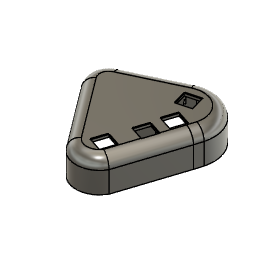
keyboard enclosure v1 (Autodesk Fusion 360 design; units mm, degrees)
Autodesk Fusion 360 part; units mm, degrees
note: some values were not read from the file. Set by a fixed rule: which face or edge a step refers to.
sketch "Sketch1" plane through (0, 0, 0) normal (0, 1, 0) x (1, 0, 0)
  line L0 (37.3318, 32.24) -> (56.8536, -27.823)
  line L1 (15.147, -72.2088) -> (-33.9094, -49.1235)
  line L2 (-42, -21) -> (0, 35)
  arc A0 (37.3318, 32.24) -> (0, 35) centre (17.782, 21.6635) ccw
  line L3 (-38.7396, -23.3195) -> (3.2, 32.6)
  arc A1 (33.646, 30.6398) -> (3.2, 32.6) centre (17.782, 21.6635) ccw
  line L4 (33.646, 30.6398) -> (53.0495, -29.0594)
  line L5 (18.0933, -69.1745) -> (-33.135, -45.0672)
  arc A2 (-38.7396, -23.3195) -> (-33.135, -45.0672) centre (-27.2324, -31.95) ccw
  arc A3 (-42, -21) -> (-33.9094, -49.1235) centre (-27.3274, -32.0045) ccw
  arc A4 (18.0933, -69.1745) -> (55.1557, -35.5397) centre (29.6328, -44.6529) ccw
  arc A5 (15.147, -72.2088) -> (59.1557, -35.5327) centre (28.6034, -43.6139) ccw
  line L6 (56.8536, -27.823) -> (59.1557, -35.5327)
  line L7 (53.0495, -29.0594) -> (55.1557, -35.5397)
  line L8 (52.453, -53.0201) -> (43.8544, -53.0201) construction
  line L9 (43.8544, -53.0201) -> (43.8544, -43.0201) construction
  line L10 (43.8544, -43.0201) -> (52.453, -43.0201) construction
  line L11 (52.453, -43.0201) -> (52.453, -53.0201) construction
  line L12 (17.453, -53.0201) -> (26.0516, -53.0201) construction
  line L13 (26.0516, -53.0201) -> (26.0516, -43.0201) construction
  line L14 (26.0516, -43.0201) -> (17.453, -43.0201) construction
  line L15 (17.453, -43.0201) -> (17.453, -53.0201) construction
  line L16 (19.8928, 4.2595) -> (7.5092, -13.426) construction
  line L17 (7.5092, -13.426) -> (-13.2972, 1.1429) construction
  line L18 (-13.2972, 1.1429) -> (-0.9137, 18.8283) construction
  line L19 (-0.9137, 18.8283) -> (19.8928, 4.2595) construction
  circle A6 centre (-0.9137, 18.8283) radius 1.25
  circle A7 centre (19.8928, 4.2595) radius 1.25
  circle A8 centre (-13.2972, 1.1429) radius 1.25
  circle A9 centre (7.5092, -13.426) radius 1.25
  point P0 (20.4966, 21.6635)
  point P1 (31.9109, -7.9188)
  point P2 (37.3318, -27.3652)
  point P3 (27.6914, -52.5189)
  point P4 (17.5, 42)
  point P5 (47.0927, -4.6835)
  point P6 (33.5812, -73.0892)
  point P7 (-42.8158, -37.0751)
  dimension "d55" = 4
  dimension "d56" = 4
  dimension "d70" = 21.59
  dimension "d71" = 25.4
  dimension "d72" = 2.5
  dimension "d73" = 2.5
  dimension "d74" = 2.5
  dimension "d75" = 2.5
  text T0 "v1" font "Arial" height 10 align ink ink in box 0 x 0 at (52.453, -53.0201) x (-1, 0) y (0, 1) spacing 1 kerned height is em
  text T1 "v1" font "Arial" height 10 align ink ink in box 0 x 0 at (17.453, -53.0201) x (1, 0) y (0, 1) spacing 1 height is em
  constraint tangent L2 A0
  constraint parallel L2 L3
  constraint concentric A0 A1
  constraint parallel L0 L4
  constraint tangent L3 A1
  constraint tangent L3 A2
  constraint tangent L2 A3
  constraint tangent L5 A4
  constraint tangent L1 A5
  constraint parallel L4 L7
  constraint perpendicular L8 L9
  constraint parallel L8 L10
  constraint parallel L9 L11
  constraint perpendicular L12 L13
  constraint parallel L12 L14
  constraint parallel L13 L15
  constraint coincident L18.end L19.start
  constraint coincident L16.start L19.end
  constraint coincident L17.end L18.start
  constraint coincident L16.end L17.start
  measures "d55" distance of L1 L5
  measures "d56" distance of A4.end A5.end
  measures "d70" distance of L16.start L16.end
  measures "d71" distance of L16.start L18.end
  measures "d72" diameter of A6
  measures "d73" diameter of A7
  measures "d74" diameter of A8
  measures "d75" diameter of A9
extrude "Extrude1" add sketch "Sketch1" along normal blind 30 contours L0 L1 L2 A0 A3 A5 L6 | L3 A1 L4 L5 A2 A4 L7 | A6 | A7 | A8 | A9 makes body 1
sketch "Sketch2" plane through (-25.0736, 0, 53.2816) normal (-0.425796, 0, 0.904819) x (0.904819, 0, 0.425796)
  line L0 (-9.7653, 0) -> (44.4515, 0)
  line L1 (44.4515, 30) -> (-9.7653, 30)
  line L2 (-7.9037, 17.6353) -> (-7.0737, 17.6353) construction
  line L3 (2.6065, 7.5699) -> (2.6065, 6.7399) construction
  line L4 (6.9063, 17.6353) -> (7.7363, 17.6353) construction
  line L5 (-7.0737, 7.5699) -> (-7.0737, 21.5499)
  line L6 (7.7363, 6.7399) -> (-7.9037, 6.7399)
  line L7 (-7.9037, 22.3799) -> (7.7363, 22.3799)
  line L8 (6.9063, 7.5699) -> (-7.0737, 7.5699)
  line L9 (6.9063, 21.5499) -> (6.9063, 7.5699)
  line L10 (7.7363, 22.3799) -> (7.7363, 6.7399)
  line L11 (-7.0737, 21.5499) -> (6.9063, 21.5499)
  line L12 (1.5152, 22.3799) -> (1.5152, 21.5499) construction
  line L13 (-7.9037, 6.7399) -> (-7.9037, 22.3799)
  line L14 (44.4515, 0) -> (44.4515, 30)
  line L15 (-9.7653, 30) -> (-9.7653, 0)
  point P0 (0, 15)
  dimension "d46" = 13.98
  dimension "d47" = 13.98
  dimension "d48" = 15.64
  dimension "d49" = 15.64
  constraint horizontal L11
  constraint vertical L9
  constraint horizontal L8
  constraint vertical L5
  constraint horizontal L7
  constraint vertical L10
  constraint horizontal L6
  constraint vertical L13
  constraint coincident L12.start L7
  constraint coincident L12.end L11
  constraint perpendicular L11 L12
  constraint coincident L3.start L8
  constraint coincident L3.end L6
  constraint perpendicular L3 L6
  constraint equal L3 L12
  constraint coincident L2.start L13
  constraint coincident L2.end L5
  constraint perpendicular L2 L5
  constraint coincident L4.start L9
  constraint coincident L4.end L10
  constraint perpendicular L4 L10
  constraint equal L2 L4
  measures "d46" distance of L5.end L9.start
  measures "d47" distance of L5.end L5.start
  measures "d48" distance of L6.end L7.start
  measures "d49" distance of L7.start L7.end
sketch "Sketch3" plane through (0, 0, 0) normal (0, 1, 0) x (1, 0, 0)
  line L0 (196.83, 143.17) -> (210.81, 143.17)
  line L1 (210.81, 143.17) -> (210.81, 129.19)
  line L2 (210.81, 129.19) -> (196.83, 129.19)
  line L3 (196.83, 129.19) -> (196.83, 143.17)
  line L4 (196, 144) -> (211.64, 144)
  line L5 (211.64, 144) -> (211.64, 128.36)
  line L6 (211.64, 128.36) -> (196, 128.36)
  line L7 (196, 128.36) -> (196, 144)
  line L8 (205.4189, 144) -> (205.4189, 143.17) construction
  line L9 (206.5102, 129.19) -> (206.5102, 128.36) construction
  line L10 (196, 139.2554) -> (196.83, 139.2554) construction
  line L11 (210.81, 139.2554) -> (211.64, 139.2554) construction
  line L12 (13.4768, 22.0727) -> (14.2661, 22.3292) construction
  line L13 (12.0106, 26.5851) -> (26.8851, 31.4181)
  line L14 (27.5619, 26.6492) -> (28.3513, 26.9057) construction
  line L15 (20.9685, 29.4957) -> (21.225, 28.7063) construction
  line L16 (13.0565, 26.0522) -> (26.3522, 30.3722)
  line L17 (17.3765, 12.7564) -> (13.0565, 26.0522)
  line L18 (31.7182, 16.5436) -> (16.8436, 11.7105)
  line L19 (26.583, 15.7478) -> (26.8394, 14.9584) construction
  line L20 (26.3522, 30.3722) -> (30.6723, 17.0765)
  line L21 (30.6723, 17.0765) -> (17.3765, 12.7564)
  line L22 (26.8851, 31.4181) -> (31.7182, 16.5436)
  line L23 (16.8436, 11.7105) -> (12.0106, 26.5851)
  line L24 (26.583, 15.7478) -> (26.8394, 14.9584) construction
  line L25 (13.4768, 22.0727) -> (14.2661, 22.3292) construction
  line L26 (12.0106, 26.5851) -> (26.8851, 31.4181)
  line L27 (26.8851, 31.4181) -> (31.7182, 16.5436)
  line L28 (20.9685, 29.4957) -> (21.225, 28.7063) construction
  line L29 (30.6723, 17.0765) -> (17.3765, 12.7564)
  line L30 (16.8436, 11.7105) -> (12.0106, 26.5851)
  line L31 (13.0565, 26.0522) -> (26.3522, 30.3722)
  line L32 (31.7182, 16.5436) -> (16.8436, 11.7105)
  line L33 (26.3522, 30.3722) -> (30.6723, 17.0765)
  line L34 (17.3765, 12.7564) -> (13.0565, 26.0522)
  line L35 (27.5619, 26.6492) -> (28.3513, 26.9057) construction
  line L36 (27.7094, -16.9369) -> (22.8764, -2.0624)
  line L37 (37.2181, 1.7248) -> (41.5381, -11.571)
  line L38 (41.5381, -11.571) -> (28.2423, -15.8911)
  line L39 (37.7509, 2.7706) -> (42.584, -12.1039)
  line L40 (28.2423, -15.8911) -> (23.9223, -2.5953)
  line L41 (23.9223, -2.5953) -> (37.2181, 1.7248)
  line L42 (42.584, -12.1039) -> (27.7094, -16.9369)
  line L43 (22.8764, -2.0624) -> (37.7509, 2.7706)
  line L44 (43.3798, -23.6452) -> (44.1692, -23.3887) construction
  line L45 (33.1944, -37.538) -> (28.8744, -24.2422)
  line L46 (29.2947, -28.2217) -> (30.084, -27.9652) construction
  line L47 (42.1701, -19.9222) -> (46.4902, -33.218)
  line L48 (43.3798, -23.6452) -> (44.1692, -23.3887) construction
  line L49 (36.7864, -20.7988) -> (37.0429, -21.5881) construction
  line L50 (42.703, -18.8763) -> (47.536, -33.7509)
  line L51 (47.536, -33.7509) -> (32.6615, -38.5839)
  line L52 (27.8285, -23.7094) -> (42.703, -18.8763)
  line L53 (47.536, -33.7509) -> (32.6615, -38.5839)
  line L54 (28.8744, -24.2422) -> (42.1701, -19.9222)
  line L55 (46.4902, -33.218) -> (33.1944, -37.538)
  line L56 (36.7864, -20.7988) -> (37.0429, -21.5881) construction
  line L57 (33.1944, -37.538) -> (28.8744, -24.2422)
  line L58 (42.703, -18.8763) -> (47.536, -33.7509)
  line L59 (28.8744, -24.2422) -> (42.1701, -19.9222)
  line L60 (32.6615, -38.5839) -> (27.8285, -23.7094)
  line L61 (27.8285, -23.7094) -> (42.703, -18.8763)
  line L62 (42.4008, -34.5467) -> (42.6573, -35.336) construction
  line L63 (29.2947, -28.2217) -> (30.084, -27.9652) construction
  line L64 (42.1701, -19.9222) -> (46.4902, -33.218)
  line L65 (46.4902, -33.218) -> (33.1944, -37.538)
  line L66 (32.6615, -38.5839) -> (27.8285, -23.7094)
  line L67 (42.4008, -34.5467) -> (42.6573, -35.336) construction
  line L68 (33.7721, -61.286) -> (18.6793, -57.1854)
  line L69 (18.6793, -57.1854) -> (22.7799, -42.0925)
  line L70 (37.8728, -46.1931) -> (33.7721, -61.286)
  line L71 (22.7799, -42.0925) -> (37.8728, -46.1931)
  line L72 (33.1888, -60.2674) -> (19.6979, -56.602)
  line L73 (19.6979, -56.602) -> (23.3633, -43.1111)
  line L74 (36.8542, -46.7765) -> (33.1888, -60.2674)
  line L75 (23.3633, -43.1111) -> (36.8542, -46.7765)
  dimension "d3" = 13.98
  dimension "d4" = 13.98
  dimension "d5" = 15.64
  dimension "d6" = 15.64
  dimension "d9" = 13.98
  dimension "d10" = 13.98
  dimension "d11" = 15.64
  dimension "d12" = 15.64
  dimension "d13" = 13.98
  dimension "d14" = 13.98
  dimension "d15" = 15.64
  dimension "d16" = 15.64
  dimension "d19" = 15.64
  dimension "d20" = 15.64
  dimension "d21" = 13.98
  dimension "d22" = 13.98
  dimension "d25" = 13.98
  dimension "d26" = 13.98
  dimension "d27" = 15.64
  dimension "d28" = 15.64
  dimension "d29" = 13.98
  dimension "d30" = 13.98
  dimension "d31" = 15.64
  dimension "d32" = 15.64
  dimension "d33" = 13.98
  dimension "d34" = 13.98
  dimension "d35" = 15.64
  dimension "d36" = 15.64
  constraint horizontal L0
  constraint vertical L1
  constraint horizontal L2
  constraint vertical L3
  constraint horizontal L4
  constraint vertical L5
  constraint horizontal L6
  constraint vertical L7
  constraint coincident L4 L8.start
  constraint coincident L0 L8.end
  constraint perpendicular L0 L8
  constraint coincident L2 L9.start
  constraint coincident L6 L9.end
  constraint perpendicular L6 L9
  constraint equal L8 L9
  constraint coincident L7 L10.start
  constraint coincident L3 L10.end
  constraint perpendicular L3 L10
  constraint coincident L1 L11.start
  constraint coincident L5 L11.end
  constraint perpendicular L5 L11
  constraint equal L10 L11
  constraint coincident L15.start L13
  constraint coincident L15.end L16
  constraint perpendicular L15 L16
  constraint coincident L19.start L21
  constraint coincident L19.end L18
  constraint perpendicular L18 L19
  constraint equal L15 L19
  constraint coincident L12.start L23
  constraint coincident L12.end L17
  constraint perpendicular L12 L17
  constraint coincident L14.start L20
  constraint coincident L14.end L22
  constraint perpendicular L14 L22
  constraint equal L12 L14
  constraint coincident L15.start L26
  constraint coincident L15.end L31
  constraint perpendicular L28 L31
  constraint coincident L19.start L29
  constraint coincident L19.end L32
  constraint perpendicular L24 L32
  constraint equal L24 L28
  constraint coincident L12.start L30
  constraint coincident L12.end L34
  constraint perpendicular L25 L34
  constraint coincident L14.start L33
  constraint coincident L14.end L27
  constraint perpendicular L27 L35
  constraint equal L25 L35
  constraint coincident L49.start L52
  constraint coincident L49.end L54
  constraint perpendicular L49 L54
  constraint coincident L62.start L65
  constraint coincident L62.end L51
  constraint perpendicular L51 L62
  constraint equal L49 L62
  constraint coincident L46.start L66
  constraint coincident L46.end L57
  constraint perpendicular L57 L63
  constraint coincident L44.start L64
  constraint coincident L44.end L58
  constraint perpendicular L48 L58
  constraint equal L48 L63
  constraint coincident L49.start L61
  constraint coincident L49.end L59
  constraint perpendicular L56 L59
  constraint coincident L62.start L55
  constraint coincident L62.end L53
  constraint perpendicular L53 L67
  constraint equal L56 L67
  constraint coincident L46.start L60
  constraint coincident L46.end L45
  constraint perpendicular L45 L46
  constraint coincident L44.start L47
  constraint coincident L44.end L50
  constraint perpendicular L44 L50
  constraint equal L44 L46
  measures "d3" distance of L0.start L0.end
  measures "d4" distance of L0.start L2.end
  measures "d5" distance of L4.start L6.end
  measures "d6" distance of L4.start L4.end
  measures "d9" distance of L16.start L16.end
  measures "d10" distance of L16.start L17.start
  measures "d11" distance of L18.end L13.start
  measures "d12" distance of L13.start L13.end
  measures "d13" distance of L16.start L16.end
  measures "d14" distance of L16.start L17.start
  measures "d15" distance of L18.end L13.start
  measures "d16" distance of L13.start L13.end
  measures "d19" distance of L36.start L36.end
  measures "d20" distance of L36.end L39.start
  measures "d21" distance of L37.start L40.end
  measures "d22" distance of L38.end L40.end
  measures "d25" distance of L47.start L45.end
  measures "d26" distance of L45.end L45.start
  measures "d27" distance of L52.start L51.end
  measures "d28" distance of L50.start L52.start
  measures "d29" distance of L45.end L47.start
  measures "d30" distance of L45.end L45.start
  measures "d31" distance of L52.start L51.end
  measures "d32" distance of L50.start L52.start
  measures "d33" distance of L74.start L73.end
  measures "d34" distance of L72.end L73.end
  measures "d35" distance of L69.end L68.end
  measures "d36" distance of L70.start L69.end
extrude "Extrude2" cut sketch "Sketch1" along normal blind 26 contours L3 A1 L4 L5 A2 A4 L7 | A6 | A7 | A8 | A9 bodies 1
split_face "SplitFace1" 1 faces at (4.9512, 30, 4.6077) by curves path "Sketch3" along L21 L17 L16 L20 on bodies 1
extrude "Extrude3" cut 1 faces at (20.3684, 30, -18.6284) along direction (0, -1, 0) blind 80 on bodies 1 bodies 1
split_face "SplitFace2" 1 faces at (-0.462, 30, 36.192) by curves path "Sketch3" along L37 L38 L40 L41 on bodies 1
split_face "SplitFace3" 1 faces at (3.16, 30, 45.7411) by curves path "Sketch3" along L64 L65 L57 L54 on bodies 1
split_face "SplitFace4" 1 faces at (4.8107, 30, 52.9568) by curves path "Sketch3" along L75 L74 L72 L73 on bodies 1
extrude "Extrude4" cut 3 faces at (34.2261, 30, 4.1472) (40.6182, 30, 30.2261) (25.4166, 30, 53.3268) along direction (0, -1, 0) blind 70 on bodies 1 bodies 1
split_face "SplitFace5" 1 faces at (-6.0544, 26, -7.3456) by curves path "Sketch3" along L27 L32 L30 L26 on bodies 1
split_face "SplitFace6" 1 faces at (-6.232, 26, -6.997) by curves path "Sketch3" along L39 L42 L36 L43 on bodies 1
split_face "SplitFace7" 1 faces at (4.111, 26, 27.7892) by curves path "Sketch3" along L53 L60 L61 L50 on bodies 1
split_face "SplitFace8" 1 faces at (-6.232, 26, -6.997) by curves path "Sketch3" along L68 L69 L71 L70 on bodies 1
extrude "Extrude5" cut 4 faces at (21.9794, 26, -13.6702) (37.2772, 26, 13.5373) (42.2293, 26, 35.1842) (28.0053, 26, 43.7989) along direction (0, 1, 0) blind 3 on bodies 1 bodies 1
extrude "Extrude6" cut sketch "Sketch2" against normal blind 31 contours L5 L8 L9 L11 bodies 1
split_face "SplitFace9" 1 faces at (6.3551, 11.19, 63.6507) by curves path "Sketch2" along L10 L6 L13 L7 on bodies 1
extrude "Extrude7" cut 1 faces at (-21.3379, 22.1032, 50.6187) along direction (-0.425796, 0, 0.904819) blind 3 on bodies 1 bodies 1
fillet "Fillet1" radius 10 7 edges at (19.4208, 30, -43.8305) (-21, 30, -7) (-44.9533, 30, 37.0751) (-9.3812, 30, 60.6662) (48.8359, 30, 67.8913) (47.0927, 30, -2.2085) (58.0047, 30, 31.6779) on bodies 1
extrude "Extrude8" add sketch "Sketch1" against normal blind 4 separate body contours L0 L1 L2 A0 A3 A5 L6 | L3 A1 L4 L5 A2 A4 L7 | A6 | A7 | A8 | A9 makes body 2
extrude "Extrude14" add sketch "Sketch1" along normal blind 1 contours L3 A1 L4 L5 A2 A4 L7 bodies 2
move_face "OffsetFaces1" offset -0.8 6 faces at (40.8159, 0.3333, -8.58) (3.7325, 0.6667, -33.2761) (-24.7598, 0.3333, 4.6797) (-39.8484, 0.6667, 38.8592) (1.0172, 0.3333, 61.1388) (48.8075, 0.6667, 63.805) on bodies 2
sketch "Sketch4" plane through (-16.8, 0, -12.6) normal (-0.8, 0, -0.6) x (-0.6, 0, 0.8)
  line L0 (42, 20) -> (-28, 20)
  line L1 (-28, 20) -> (-28, 0)
  line L2 (-28, 0) -> (42, 0)
  line L3 (42, 0) -> (42, 20)
  circle A0 centre (-25.2593, 0) radius 2
  dimension "d59" = 4
  constraint coincident L2 A0.centre
  measures "d59" diameter of A0
extrude "Extrude9" cut sketch "Sketch4" against normal blind 4.1 contours L2 A0 | L2 A0 bodies 1 2
sketch "Sketch5" plane through (0, 0, 0) normal (0, 1, 0) x (1, 0, 0)
  line L0 (2.75, 32) -> (3.8, 33.4)
  line L1 (3.8, 33.4) -> (6.8342, 31.1244)
  line L2 (6.8342, 31.1244) -> (2.6395, 25.5316)
  line L3 (2.6395, 25.5316) -> (-0.3844, 27.7995)
  line L4 (-0.3844, 27.7995) -> (2.75, 32)
  constraint perpendicular L0 L1
  constraint perpendicular L1 L2
  constraint perpendicular L2 L3
extrude "Extrude10" cut sketch "Sketch5" against normal blind 3.8 from surface at 1 bodies 2
chamfer "Chamfer1" distance 3.8 angle 45 1 edges at (4.7369, 1, -28.328) on bodies 2
extrude "Extrude11" cut sketch "Sketch1" along normal blind 1 from surface at 26 text T0 bodies 1
extrude "Extrude12" cut sketch "Sketch1" against normal blind 1 from surface at 1 text T1 bodies 2
extrude "Extrude13" add sketch "Sketch1" against normal blind 12.5 from surface at 26 contours A6 | A7 | A8 | A9 bodies 1
draft "Draft1" angle 3 neutral plane through (0, 26, 0) pull (0, -1, 0) 4 faces at (-12.0534, 21.8333, -1.0184) (8.753, 21.8333, 13.5504) (21.1366, 21.8333, -4.135) (0.3301, 21.8333, -18.7039) on bodies 1
mirror "Mirror1" about plane through (0, 0, 0) normal (0, 0, 1) of bodies 1 makes body 3
mirror "Mirror2" about plane through (0, 0, 0) normal (0, 0, 1) of bodies 2 makes body 4
copy_body "Body->Comp1" bodies 1 removing the originals makes body 5 in component "left"
copy_body "CutPasteBodies1" bodies 2 removing the originals makes body 6 in component "left"
copy_body "Body->Comp2" bodies 3 removing the originals makes body 7 in component "right"
copy_body "CutPasteBodies1'" bodies 4 removing the originals makes body 8 in component "right"
delete_face "DeleteFace1" 1 faces at (8.3989, 25.3056, -14.2514) on bodies 7 in component "right"
delete_face "DeleteFace2" 1 faces at (-12.6904, 25.3056, 2.1939) on bodies 7 in component "right"
delete_face "DeleteFace3" 1 faces at (-0.0241, 25.3056, 19.6538) on bodies 7 in component "right"
delete_face "DeleteFace4" 1 faces at (19.8021, 25.3056, 5.4697) on bodies 7 in component "right"
delete_face "DeleteFace5" 1 faces at (8.7577, 0.6667, -13.4883) on bodies 8 in component "right"
delete_face "DeleteFace6" 1 faces at (21.1412, 0.6667, 4.1972) on bodies 8 in component "right"
delete_face "DeleteFace7" 1 faces at (-12.0488, 0.6667, 1.0805) on bodies 8 in component "right"
delete_face "DeleteFace8" 1 faces at (0.3347, 0.6667, 18.766) on bodies 8 in component "right"
move_face "OffsetFaces1'" offset -3 1 faces at (7.0569, -0.2664, 30.9573) on bodies 8 in component "right"
move_face "OffsetFaces2" offset -4 1 faces at (0.8335, -1.8664, 26.8861) on bodies 8 in component "right"
move_face "OffsetFaces3" offset -3 2 faces at (5.836, -2.7995, 29.7934) (4.9694, -1.8662, 27.0829) on bodies 8 in component "right"
move_face "OffsetFaces4" offset 0.5 1 faces at (6.1369, -2.8, 27.5886) on bodies 8 in component "right"
sketch "Sketch1 (2)" plane through (-23.3704, 0, -49.6623) normal (0.425796, 0, 0.904819) x (0.904819, 0, -0.425796) in component "right"
  line L0 (7.7363, 22.3799) -> (7.7363, 6.7399)
  line L1 (7.7363, 6.7399) -> (-7.9037, 6.7399)
  line L2 (-7.9037, 6.7399) -> (-7.9037, 22.3799)
  line L3 (-7.9037, 22.3799) -> (7.7363, 22.3799)
  line L4 (-10.7918, 0) -> (45.8254, 0)
  line L5 (45.8254, 0) -> (45.8254, 26)
  line L6 (45.8254, 26) -> (-10.7918, 26)
  line L7 (-10.7918, 26) -> (-10.7918, 0)
  line L8 (7.7363, 22.3799) -> (7.7363, 6.7399)
  line L9 (7.7363, 6.7399) -> (-7.9037, 6.7399)
  line L10 (-7.9037, 6.7399) -> (-7.9037, 22.3799)
  line L11 (-7.9037, 22.3799) -> (7.7363, 22.3799)
  line L12 (-10.7918, 0) -> (45.8254, 0)
  line L13 (45.8254, 0) -> (45.8254, 26)
  line L14 (45.8254, 26) -> (-10.7918, 26)
  line L15 (-10.7918, 26) -> (-10.7918, 0)
  line L16 (-29.4398, 0) -> (-9.7653, 0)
  line L17 (44.4515, 0) -> (-9.7653, 0)
  line L18 (44.4515, 0) -> (76.0545, 0)
  line L19 (66.0545, 30) -> (44.4515, 30)
  line L20 (44.4515, 30) -> (-10.2003, 30)
  line L21 (-10.2003, 30) -> (-19.4398, 30)
  line L22 (-29.4398, 20) -> (-29.4398, 0)
  line L23 (76.0545, 20) -> (76.0545, 0)
  arc A0 (76.0545, 20) -> (66.0545, 30) centre (66.0545, 20) ccw
  arc A1 (-19.4398, 30) -> (-29.4398, 20) centre (-19.4398, 20) ccw
  line L24 (27.2493, 0) -> (27.2493, 10.6) construction
  line L25 (31.2493, 12.19) -> (23.2493, 12.19)
  line L26 (23.2493, 12.19) -> (23.2493, 9.01)
  line L27 (23.2493, 9.01) -> (31.2493, 9.01)
  line L28 (31.2493, 9.01) -> (31.2493, 12.19)
  line L29 (31.2493, 12.19) -> (23.2493, 9.01) construction
  line L30 (23.2493, 12.19) -> (31.2493, 9.01) construction
  line L31 (36.7493, 13.6) -> (17.7493, 13.6)
  line L32 (17.7493, 13.6) -> (17.7493, 7.6)
  line L33 (17.7493, 7.6) -> (36.7493, 7.6)
  line L34 (36.7493, 7.6) -> (36.7493, 13.6)
  line L35 (36.7493, 13.6) -> (17.7493, 7.6) construction
  line L36 (17.7493, 13.6) -> (36.7493, 7.6) construction
  line L37 (15.4242, 13.5209) -> (38.4242, 13.5209)
  line L38 (38.4242, 13.5209) -> (38.4242, 25.9559)
  line L39 (38.4242, 25.9559) -> (15.4242, 25.9559)
  line L40 (15.4242, 25.9559) -> (15.4242, 13.5209)
  line L41 (31.2493, 9.01) -> (31.2493, 12.19)
  line L42 (31.2493, 12.19) -> (23.2493, 12.19)
  line L43 (23.2493, 12.19) -> (23.2493, 9.01)
  line L44 (23.2493, 9.01) -> (31.2493, 9.01)
  line L45 (25.6792, 20.3031) -> (25.6792, 12.3031)
  line L46 (25.6792, 12.3031) -> (28.8592, 12.3031)
  line L47 (28.8592, 12.3031) -> (28.8592, 20.3031)
  line L48 (28.8592, 20.3031) -> (25.6792, 20.3031)
  point P0 (27.2493, 10.6)
  point P1 (27.2493, 10.6)
  dimension "d131" = 10.6
  dimension "d132" = 8
  dimension "d133" = 3.18
  dimension "d134" = 19
  dimension "d135" = 6
  dimension "d136" = 23
  dimension "d144" = 8
  dimension "d145" = 3.18
  dimension "d146" = 8
  dimension "d147" = 3.18
  constraint coincident L4 L24.start
  constraint perpendicular L17 L24
  constraint perpendicular L25 L26
  constraint parallel L25 L27
  constraint parallel L26 L28
  constraint horizontal L25
  constraint coincident L29 P1
  constraint coincident L30 P1
  constraint coincident P1 P0
  constraint perpendicular L31 L32
  constraint parallel L31 L33
  constraint parallel L32 L34
  constraint horizontal L31
  constraint coincident L35 P1
  constraint coincident L36 P1
  constraint horizontal L37
  constraint vertical L38
  constraint horizontal L39
  constraint vertical L40
  constraint perpendicular L42 L43
  constraint parallel L42 L44
  constraint parallel L41 L43
  constraint horizontal L42
  constraint perpendicular L47 L48
  constraint parallel L45 L47
  constraint parallel L46 L48
  measures "d131" distance of L24.start P1
  measures "d132" distance of L26.end L27.end
  measures "d133" distance of L25.end L26.end
  measures "d134" distance of L32.end L33.end
  measures "d135" distance of L31.end L32.end
  measures "d136" distance of L37.start L37.end
  measures "d144" distance of L26.end L27.end
  measures "d145" distance of L25.end L26.end
  measures "d146" distance of L45.end L45.start
  measures "d147" distance of L47.end L45.start
extrude "Extrude8'" cut sketch "Sketch1 (2)" against normal blind 9 contours L31 L37 L45 L47 | L31 L45 L47 L48 | L37 L45 L46 L47 bodies 7 in component "right"
extrude "Extrude9'" cut sketch "Sketch1 (2)" against normal up to surface (1 mm away) contours L25 L26 L27 L28 L41 L42 L43 L44 | L31 L34 L37 L47 | L31 L32 L34 L37 L38 L39 L40 L45 L47 L48 | L31 L37 L45 L47 | L31 L45 L47 L48 | L32 L33 L34 L37 L45 L46 L47 | L31 L32 L37 L45 | L37 L45 L46 L47 bodies 7 in component "right"
chamfer "Chamfer6" distance 1 angle 45 1 edges at (0.5653, 25.9559, -62.0313) on bodies 7 in component "right"
move_face "OffsetFaces6" offset -1.1 1 faces at (-6.0458, 19.5934, -58.9202) on bodies 7 in component "right"
chamfer "Chamfer7" distance 2.1 angle 45 3 edges at (-8.3624, 13.5209, -56.7248) (1.2853, 7.6, -61.2649) (10.6388, 13.5209, -65.6666) on bodies 7 in component "right"
sketch "Sketch2 (2)" plane through (0, 1, 0) normal (0, 1, 0) x (-1, 0, 0) in component "right"
  line L0 (-26.0616, -53.0001) -> (-26.0616, -45.8126)
  line L1 (-26.0616, -45.8126) -> (-25.4952, -45.8126)
  spline S0 degree 3 poles (-24.714, -46.7697) (-24.8662, -46.6278) (-25.0185, -46.486) (-25.2831, -46.1667) (-25.376, -46.0116) (-25.4952, -45.8126) knots 0 0 0 0 0.062422 0.062422 0.125715 0.125715 0.125715 0.125715
  spline S1 degree 3 poles (-23.4249, -47.6095) (-23.655, -47.4928) (-23.885, -47.3761) (-24.3154, -47.0967) (-24.506, -46.9403) (-24.714, -46.7697) knots 0 0 0 0 0.077391 0.077391 0.15487 0.15487 0.15487 0.15487
  line L2 (-23.4249, -47.6095) -> (-23.4249, -48.4591)
  spline S2 degree 3 poles (-24.3502, -48.005) (-24.2008, -48.0906) (-24.0514, -48.1761) (-23.7418, -48.3292) (-23.6011, -48.3869) (-23.4249, -48.4591) knots 0 0 0 0 0.051652 0.051652 0.103847 0.103847 0.103847 0.103847
  spline S3 degree 3 poles (-25.1827, -47.3995) (-25.0391, -47.5245) (-24.9243, -47.6244) (-24.6446, -47.8262) (-24.4974, -47.9156) (-24.3502, -48.005) knots 0 0 0 0 0.057103 0.057103 0.113619 0.113619 0.113619 0.113619
  line L3 (-25.1827, -47.3995) -> (-25.1827, -53.0001)
  line L4 (-25.1827, -53.0001) -> (-26.0616, -53.0001)
  line L5 (-19.4357, -53.0001) -> (-20.256, -53.0001)
  line L6 (-20.256, -53.0001) -> (-22.2189, -47.8146)
  line L7 (-22.2189, -47.8146) -> (-21.3155, -47.8146)
  line L8 (-21.3155, -47.8146) -> (-20.1632, -50.9786)
  spline S4 degree 3 poles (-19.8361, -51.965) (-19.8919, -51.78) (-19.9356, -51.6356) (-20.0458, -51.3047) (-20.1045, -51.1417) (-20.1632, -50.9786) knots 0 0 0 0 0.057966 0.057966 0.11515 0.11515 0.11515 0.11515
  spline S5 degree 3 poles (-19.504, -50.9201) (-19.5656, -51.0969) (-19.6242, -51.2653) (-19.7348, -51.6137) (-19.7854, -51.7893) (-19.8361, -51.965) knots 0 0 0 0 0.05617 0.05617 0.112321 0.112321 0.112321 0.112321
  line L9 (-19.504, -50.9201) -> (-18.3907, -47.8146)
  line L10 (-18.3907, -47.8146) -> (-17.463, -47.8146)
  line L11 (-17.463, -47.8146) -> (-19.4357, -53.0001)
  line L12 (2.1546, 24.1272) -> (-6.6737, 17.506)
  line L13 (-6.6737, 17.506) -> (-15.0683, 28.6988)
  line L14 (-15.0683, 28.6988) -> (-6.6122, 35.0408)
  arc A0 (-6.6122, 35.0408) -> (-32.9103, 30.3151) centre (-17.782, 21.6635) ccw
  line L15 (-32.9103, 30.3151) -> (-54.3985, -35.7979)
  arc A1 (-54.3985, -35.7979) -> (-18.4339, -68.4507) centre (-29.6328, -44.6529) ccw
  line L16 (-18.4339, -68.4507) -> (32.8006, -44.3404)
  arc A2 (32.8006, -44.3404) -> (38.0996, -23.7995) centre (27.2324, -31.95) ccw
  line L17 (38.0996, -23.7995) -> (2.1546, 24.1272)
  line L18 (-17.2949, -67.9147) -> (-30.3728, -22.945)
  line L19 (-30.3728, -22.945) -> (-4.4906, -11.6121)
  line L20 (-4.4906, -11.6121) -> (13.7627, -53.2994)
  line L21 (13.7627, -53.2994) -> (-17.2949, -67.9147)
  line L22 (10.1266, -55.8946) -> (-10.7021, -65.6963)
  line L23 (-10.7021, -65.6963) -> (10.1266, -55.8946)
  line L24 (9.2143, -56.3242) -> (-7.9773, -64.4143)
  line L25 (-7.9773, -64.4143) -> (9.2143, -56.3242)
  line L26 (4.01, -58.7732) -> (-3.1381, -62.137)
  line L27 (-3.1381, -62.137) -> (4.01, -58.7732)
  point P0 (10.1266, -55.8946)
  point P1 (-10.7021, -65.6963)
  point P2 (9.2143, -56.3242)
  point P3 (-7.9773, -64.4143)
  point P4 (-3.1381, -62.137)
  point P5 (4.01, -58.7732)
  constraint perpendicular L19 L20
  constraint coincident L16 L20.end
  constraint coincident L16 L18.start
extrude "Extrude1'" cut sketch "Sketch2 (2)" against normal up to surface (3 mm away) contours L5 L6 L7 L8 S4 S5 L9 L10 L11 | L16 L18 L19 L20 L21 bodies 8 in component "right"
sketch "Sketch3 (2)" plane through (0, 26, 0) normal (0, -1, 0) x (1, 0, 0) in component "right"
  arc A0 (-38.7396, -23.3195) -> (-33.135, -45.0672) centre (-27.2324, -31.95) ccw
  arc A1 (18.0933, -69.1745) -> (55.1557, -35.5397) centre (29.6328, -44.6529) ccw
  line L0 (55.1557, -35.5397) -> (33.646, 30.6398)
  arc A2 (33.646, 30.6398) -> (3.2, 32.6) centre (17.782, 21.6635) ccw
  line L1 (3.2, 32.6) -> (-38.7396, -23.3195)
  line L2 (43.8444, -45.8126) -> (44.4108, -45.8126)
  spline S0 degree 3 poles (45.192, -46.7697) (45.0398, -46.6278) (44.8875, -46.486) (44.6229, -46.1667) (44.53, -46.0116) (44.4108, -45.8126) knots 0 0 0 0 0.062422 0.062422 0.125715 0.125715 0.125715 0.125715
  spline S1 degree 3 poles (46.4811, -47.6095) (46.251, -47.4928) (46.021, -47.3761) (45.5906, -47.0967) (45.4, -46.9403) (45.192, -46.7697) knots 0 0 0 0 0.077391 0.077391 0.15487 0.15487 0.15487 0.15487
  line L3 (46.4811, -47.6095) -> (46.4811, -48.4591)
  spline S2 degree 3 poles (45.5558, -48.005) (45.7052, -48.0906) (45.8546, -48.1761) (46.1642, -48.3292) (46.3049, -48.3869) (46.4811, -48.4591) knots 0 0 0 0 0.051652 0.051652 0.103847 0.103847 0.103847 0.103847
  spline S3 degree 3 poles (44.7233, -47.3995) (44.8669, -47.5245) (44.9817, -47.6244) (45.2614, -47.8262) (45.4086, -47.9156) (45.5558, -48.005) knots 0 0 0 0 0.057103 0.057103 0.113619 0.113619 0.113619 0.113619
  line L4 (44.7233, -47.3995) -> (44.7233, -53.0001)
  line L5 (44.7233, -53.0001) -> (43.8444, -53.0001)
  line L6 (43.8444, -53.0001) -> (43.8444, -45.8126)
  line L7 (49.65, -53.0001) -> (47.6871, -47.8146)
  line L8 (47.6871, -47.8146) -> (48.5905, -47.8146)
  line L9 (48.5905, -47.8146) -> (49.7428, -50.9786)
  spline S4 degree 3 poles (50.07, -51.965) (50.0141, -51.78) (49.9704, -51.6356) (49.8602, -51.3047) (49.8015, -51.1417) (49.7428, -50.9786) knots 0 0 0 0 0.057966 0.057966 0.11515 0.11515 0.11515 0.11515
  spline S5 degree 3 poles (50.402, -50.9201) (50.3404, -51.0969) (50.2818, -51.2653) (50.1712, -51.6137) (50.1206, -51.7893) (50.07, -51.965) knots 0 0 0 0 0.05617 0.05617 0.112321 0.112321 0.112321 0.112321
  line L10 (50.402, -50.9201) -> (51.5153, -47.8146)
  line L11 (51.5153, -47.8146) -> (52.443, -47.8146)
  line L12 (52.443, -47.8146) -> (50.4703, -53.0001)
  line L13 (50.4703, -53.0001) -> (49.65, -53.0001)
  line L14 (33.7721, -61.286) -> (18.6793, -57.1854)
  line L15 (18.6793, -57.1854) -> (22.7799, -42.0925)
  line L16 (22.7799, -42.0925) -> (37.8728, -46.1931)
  line L17 (37.8728, -46.1931) -> (33.7721, -61.286)
  line L18 (47.536, -33.7509) -> (32.6615, -38.5839)
  line L19 (32.6615, -38.5839) -> (27.8285, -23.7094)
  line L20 (27.8285, -23.7094) -> (42.703, -18.8763)
  line L21 (42.703, -18.8763) -> (47.536, -33.7509)
  line L22 (37.7509, 2.7706) -> (42.584, -12.1039)
  line L23 (42.584, -12.1039) -> (27.7094, -16.9369)
  line L24 (27.7094, -16.9369) -> (22.8764, -2.0624)
  line L25 (22.8764, -2.0624) -> (37.7509, 2.7706)
  line L26 (26.8851, 31.4181) -> (31.7182, 16.5436)
  line L27 (31.7182, 16.5436) -> (16.8436, 11.7105)
  line L28 (16.8436, 11.7105) -> (12.0106, 26.5851)
  line L29 (12.0106, 26.5851) -> (26.8851, 31.4181)
  line L30 (3.7, -64.965) -> (24.3085, -21.1717)
  line L31 (24.3085, -21.1717) -> (28.1221, -22.9664)
  line L32 (28.1221, -22.9664) -> (30.2511, -18.4423)
  line L33 (30.2511, -18.4423) -> (17.6881, -12.5303)
  line L34 (17.6881, -12.5303) -> (15.5591, -17.0544)
  line L35 (24.3085, -21.1717) -> (15.5591, -17.0544)
  line L36 (-33.135, -45.0672) -> (18.0933, -69.1745)
  dimension "d118" = 48.4
  dimension "d119" = 5
  dimension "d120" = 5
  constraint perpendicular L30 L31
  constraint perpendicular L31 L32
  constraint perpendicular L32 L33
  constraint perpendicular L33 L34
  measures "d118" distance of L30.start L30.end
  measures "d119" distance of L31.end L32.end
  measures "d120" distance of L33.end L34.end
extrude "Extrude6'" add sketch "Sketch3 (2)" along normal blind 13 contours L31 L32 L33 L34 L35 bodies 7 in component "right"
component "left" placed x (1, 0, 0) y (0, 1, 0) z (0, 0, 1) at (41.5106, -11.0449, -145.824)
component "right" placed x (1, 0, 0) y (0, 1, 0) z (0, 0, 1) at (75.6992, -16.1029, 55.9954)
hidden bodies 8
named bodies: "left top", "left bottom", "right top", "right bottom"
